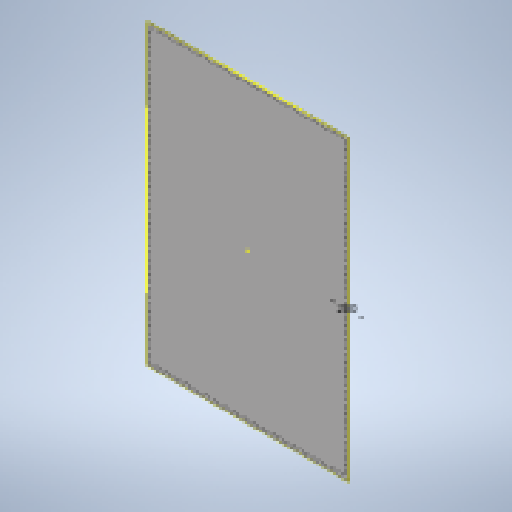
# Autodesk Inventor part: GBK bottom
Saved by Autodesk Inventor 2026.2 (Build 302298000, 298)
## iProperties
Created: 2026-04-17
Part Number: GBK bottom
Material: Generic
Document SubType Name: Sheet Metal
Designer: admin
Density: 1 g/cm^3
Sheet Metal Rule: Default_mm
Appearance: Default
Mass: 1.29377e+06 g
Surface Area: 4.31615e+06 cm^2
Volume: 1.29377e+06 cm^3
Flat Pattern Width: 1208 cm
Flat Pattern Length: 1812.6 cm
Flat Pattern Area: 2.18962e+06 cm^2
Sheet Metal Width: 12080,000 mm
Sheet Metal Length: 18126,000 mm
Sheet Metal Area: 218962080,000 mm^2
Author: admin
Autodesk Inventor part; units mm, degrees
ref_plane "YZ Plane" through (0, 0, 0) normal (1, 0, 0) x (0, 1, 0)
ref_plane "XZ Plane" through (0, 0, 0) normal (0, 1, 0) x (-1, 0, 0)
ref_plane "XY Plane" through (0, 0, 0) normal (0, 0, 1) x (1, 0, 0)
sketch "Sketch1" plane through (0, 0, 0) normal (0, 0, 1) x (1, 0, 0)
  line L0 (6040, -9063) -> (-6040, -9063)
  line L1 (-6040, -9063) -> (-6040, 9063)
  line L2 (-6040, 9063) -> (6040, 9063)
  line L3 (6040, 9063) -> (6040, -9063)
  line L4 (6040, -9063) -> (-6040, 9063) construction
  line L5 (-6040, -9063) -> (6040, 9063) construction
  point P0 (0, 0)
  dimension "d0" = 12080
  dimension "d1" = 18126
  measures "d0" distance of L1.end L2.end
  measures "d1" distance of L0.end L1.end
extrude "Plate1" add sketch "Sketch1" along normal blind 6
sketch "Эскиз7" plane through (0, 0, 6) normal (0, 0, 1) x (1, 0, 0)
  line L0 (6040, 9063) -> (6040, -9063) projected
  line L1 (-6040, 9063) -> (6040, 9063) projected
  line L2 (-6040, -9063) -> (-6040, 9063) projected
  line L3 (6040, -9063) -> (-6040, -9063) projected
  line L4 (6040, 6088) -> (6040, 9063)
  line L5 (5840, -8863) -> (5840, 8863) construction
  line L6 (5840, 8863) -> (-5840, 8863) construction
  line L7 (-5840, 8863) -> (-5840, -8863) construction
  line L8 (-5840, -8863) -> (5840, -8863) construction
  point P0 (0, 0)
  dimension "d136" = 200
  constraints: 10 end point, 3 other
  measures "d136" distance between parallel lines of L0 L5
equation "\"d2\" = Thickness"
equation "\"BendRadius\" = Thickness"
equation "\"BendReliefWidth\" = Thickness"
equation "\"BendReliefDepth\" = 0.5 * Thickness"
equation "\"CornerReliefSize\" = 4 * Thickness"
equation "\"MinimumRemnant\" = 2 * Thickness"
equation "\"TransitionRadius\" = BendRadius"
equation "\"JacobiRadiusSize\" = BendRadius"
equation "\"GapSize\" = Thickness"
equation "\"Thickness\" = 6"
body "Solid1"
